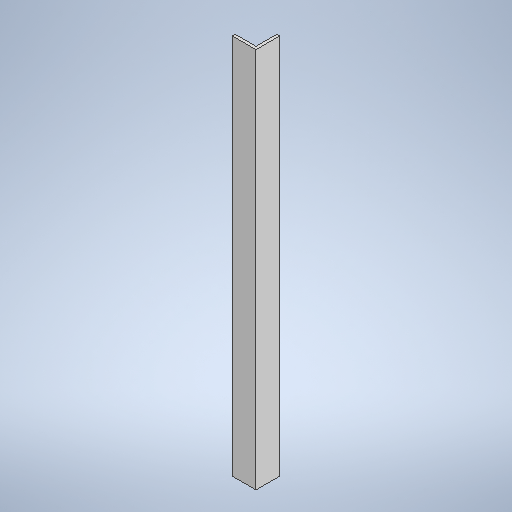
# Autodesk Inventor part: project MS angle
Saved by Autodesk Inventor 2025.2 (Build 292293000, 293)
## iProperties
Created: 2025-02-04
Part Number: project MS angle
Material: Generic
Document SubType Name: Modeling
Designer: nandu
Density: 1 g/cm^3
Appearance: Default
Author: nandu
Autodesk Inventor part; units mm, degrees
ref_plane "YZ Plane" through (0, 0, 0) normal (1, 0, 0) x (0, 1, 0)
ref_plane "XZ Plane" through (0, 0, 0) normal (0, 1, 0) x (-1, 0, 0)
ref_plane "XY Plane" through (0, 0, 0) normal (0, 0, 1) x (1, 0, 0)
sketch "Sketch1" plane through (0, 0, 0) normal (0, 1, 0) x (-1, 0, 0)
  line L0 (0, 0) -> (0, -25)
  line L1 (0, -25) -> (3, -25)
  line L2 (3, -25) -> (3, -3)
  line L3 (3, -3) -> (25, -3)
  line L4 (25, -3) -> (25, 0)
  line L5 (25, 0) -> (0, 0)
  dimension "d0" = 25
  dimension "d1" = 3
  dimension "d2" = 22
  dimension "d3" = 22
  constraints: 12 end point, 5 perpendicular, 1 vertical
  measures "d0" distance of L0.start L0.end
  measures "d1" distance of L0.end L1.end
  measures "d2" distance of L1.end L2.end
  measures "d3" distance of L2.end L3.end
extrude "Extrusion1" add sketch "Sketch1" along normal blind 400
body "Solid1"
